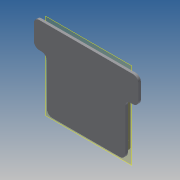
# Autodesk Inventor part: bottom plate cap
Saved by Autodesk Inventor 2013 (Build 170138000, 138)
## iProperties
Created: 2017-04-08
Part Number: bottom plate cap
Material: Generic
Document SubType Name: Modeling
Designer: employee
Density: 1 g/cm^3
Author: employee
Autodesk Inventor part; units mm, degrees
ref_plane "YZ Plane" through (0, 0, 0) normal (1, 0, 0) x (0, 1, 0)
ref_plane "XZ Plane" through (0, 0, 0) normal (0, 1, 0) x (-1, 0, 0)
ref_plane "XY Plane" through (0, 0, 0) normal (0, 0, 1) x (1, 0, 0)
ref_plane "Work Plane1" through (0, 0, 0) normal (0, 0, 1) x (1, 0, 0)
sketch "Sketch1" plane through (0, 0, 0) normal (0, 0, 1) x (1, 0, 0)
  line L0 (70, 65) -> (70, -65) projected
  arc A0 (65, -70) -> (70, -65) centre (65, -65) ccw projected
  line L1 (65, -70) -> (-65, -70) projected
  arc A1 (-70, -65) -> (-65, -70) centre (-65, -65) ccw projected
  line L2 (-70, -65) -> (-70, 65) projected
  arc A2 (-65, 70) -> (-70, 65) centre (-65, 65) ccw projected
  line L3 (-65, 70) -> (65, 70) projected
  arc A3 (70, 65) -> (65, 70) centre (65, 65) ccw projected
  arc A4 (-75, -65) -> (-65, -75) centre (-65, -65) ccw projected
  line L4 (-65, -75) -> (65, -75) projected
  arc A5 (65, -75) -> (75, -65) centre (65, -65) ccw projected
  line L5 (75, -65) -> (75, 65) projected
  arc A6 (75, 65) -> (65, 75) centre (65, 65) ccw projected
  line L6 (65, 75) -> (-65, 75) projected
  arc A7 (-65, 75) -> (-75, 65) centre (-65, 65) ccw projected
  line L7 (-75, 65) -> (-75, -65) projected
  line L8 (-65, 65) -> (-65, -65)
  line L9 (-65, -65) -> (65, -65)
  line L10 (65, -65) -> (65, 65)
  line L11 (65, 65) -> (-65, 65)
  point P0 (0, 0)
  dimension "d0" = 5
  constraints: 8 end point, 23 other
  measures "d0" distance between parallel lines of L8 L2
extrude "Extrusion1" add sketch "Sketch1" against normal blind 10 contours L0 A0 L1 A1 L2 A2 L3 A3
sketch "Sketch2" plane through (0, 0, 0) normal (0, 0, 1) x (1, 0, 0)
  line L0 (65, -65) -> (-65, -65) projected
  line L1 (70, 65) -> (70, -65) construction
  arc A0 (65, -70) -> (70, -65) centre (65, -65) ccw projected
  line L2 (65, -70) -> (-65, -70) projected
  arc A1 (-70, -65) -> (-65, -70) centre (-65, -65) ccw projected
  line L3 (-70, -65) -> (-70, 65) projected
  arc A2 (-65, 70) -> (-70, 65) centre (-65, 65) ccw projected
  line L4 (-65, 70) -> (65, 70) projected
  arc A3 (70, 65) -> (65, 70) centre (65, 65) ccw projected
  arc A4 (-75, -65) -> (-65, -75) centre (-65, -65) ccw projected
  line L5 (-65, -75) -> (65, -75) projected
  arc A5 (65, -75) -> (75, -65) centre (65, -65) ccw projected
  line L6 (75, -65) -> (75, 65) projected
  arc A6 (75, 65) -> (65, 75) centre (65, 65) ccw construction
  line L7 (65, 75) -> (-65, 75) projected
  arc A7 (-65, 75) -> (-75, 65) centre (-65, 65) ccw projected
  line L8 (-75, 65) -> (-75, -65) projected
  line L9 (-65, 75) -> (-90, 75)
  arc A8 (-90, 75) -> (-100, 65) centre (-90, 65) ccw
  line L10 (-100, 65) -> (-100, 35)
  arc A9 (-100, 35) -> (-90, 25) centre (-90, 35) ccw
  line L11 (-90, 25) -> (-85, 25)
  arc A10 (-75, 15) -> (-85, 25) centre (-85, 15) ccw
  line L12 (65, 75) -> (90, 75)
  arc A11 (100, 65) -> (90, 75) centre (90, 65) ccw
  line L13 (100, 65) -> (100, 35)
  arc A12 (90, 25) -> (100, 35) centre (90, 35) ccw
  line L14 (90, 25) -> (85, 25)
  line L15 (65, 75) -> (-65, 75)
  line L16 (-75, 15) -> (-75, -65)
  arc A13 (85, 25) -> (75, 15) centre (85, 15) ccw
  line L17 (75, 15) -> (75, -65)
  point P0 (0, 0)
  dimension "d3" = 25
  dimension "d4" = 50
  constraints: 20 tangent, 18 end point, 12 point on circle, 6 centre point, 6 equal radius, 4 perpendicular, 3 parallel, 2 collinear, 2 equal length, 2 point on line
  measures "d3" distance between parallel lines of L10 L8
  measures "d4" distance between parallel lines of L14 L12
extrude "Extrusion2" add sketch "Sketch2" along normal blind 5
sketch "Sketch3" plane through (0, 0, -10) normal (0, 0, -1) x (-1, 0, 0)
  line L0 (-70, 65) -> (-70, -65) projected
  arc A0 (-70, -65) -> (-65, -70) centre (-65, -65) ccw projected
  line L1 (-65, -70) -> (65, -70) projected
  arc A1 (65, -70) -> (70, -65) centre (65, -65) ccw projected
  line L2 (70, -65) -> (70, 65) projected
  arc A2 (70, 65) -> (65, 70) centre (65, 65) ccw projected
  line L3 (65, 70) -> (-65, 70) projected
  arc A3 (-65, 70) -> (-70, 65) centre (-65, 65) ccw projected
  line L4 (-69.5, -65) -> (-69.5, 65)
  arc A4 (-65, 69.5) -> (-69.5, 65) centre (-65, 65) ccw
  line L5 (-65, 69.5) -> (65, 69.5)
  arc A5 (69.5, 65) -> (65, 69.5) centre (65, 65) ccw
  line L6 (69.5, 65) -> (69.5, -65)
  arc A6 (65, -69.5) -> (69.5, -65) centre (65, -65) ccw
  line L7 (65, -69.5) -> (-65, -69.5)
  arc A7 (-69.5, -65) -> (-65, -69.5) centre (-65, -65) ccw
  point P0 (0, 0)
  dimension "d7" = 0.5
  constraints: 8 end point, 8 point on circle, 4 centre point, 7 other
  measures "d7" distance between parallel lines of L0 L4
extrude "Extrusion3" cut sketch "Sketch3" against normal up to surface (10 mm away)
sketch "Sketch4" plane through (-69.5, -65, -10) normal (-1, 0, 0) x (0, 0, 1)
  circle A0 centre (5, 115) radius 1.75 projected
  circle A1 centre (5, 15) radius 1.75 projected
  line L0 (-55.6, 130) -> (-55, 129.4) projected
  line L1 (-55, 129.4) -> (-15.8284, 129.4) projected
  arc A2 (-15.8284, 129.4) -> (-14.4142, 129.9858) centre (-15.8284, 131.4) ccw projected
  line L2 (-13.5858, 130.8142) -> (-14.4142, 129.9858) projected
  arc A3 (-13.5858, 130.8142) -> (-13, 132.2284) centre (-15, 132.2284) ccw projected
  line L3 (-13, 132.2284) -> (-13, 132.5) projected
  line L4 (-13, 132.5) -> (1, 132.5) projected
  line L5 (1, 130) -> (1, 132.5) projected
  line L6 (1, 130) -> (10, 130) projected
  line L7 (10, 0) -> (10, 130) projected
  line L8 (-65, 0) -> (10, 0) projected
  line L9 (-65, 130) -> (-65, 0) projected
  line L10 (-65, 130) -> (-55.6, 130) projected
  line L11 (-17.5711, 15) -> (-10.5, 7.9289) projected
  line L12 (-10.5, 7.9289) -> (-3.4289, 15) projected
  line L13 (-3.4289, 15) -> (-10.5, 22.0711) projected
  line L14 (-10.5, 22.0711) -> (-17.5711, 15) projected
  line L15 (-17.5711, 40) -> (-10.5, 32.9289) projected
  line L16 (-10.5, 32.9289) -> (-3.4289, 40) projected
  line L17 (-3.4289, 40) -> (-10.5, 47.0711) projected
  line L18 (-10.5, 47.0711) -> (-17.5711, 40) projected
  line L19 (-17.5711, 65) -> (-10.5, 57.9289) projected
  line L20 (-10.5, 57.9289) -> (-3.4289, 65) projected
  line L21 (-3.4289, 65) -> (-10.5, 72.0711) projected
  line L22 (-10.5, 72.0711) -> (-17.5711, 65) projected
  line L23 (-17.5711, 90) -> (-10.5, 82.9289) projected
  line L24 (-10.5, 82.9289) -> (-3.4289, 90) projected
  line L25 (-3.4289, 90) -> (-10.5, 97.0711) projected
  line L26 (-10.5, 97.0711) -> (-17.5711, 90) projected
  line L27 (-17.5711, 115) -> (-10.5, 107.9289) projected
  line L28 (-10.5, 107.9289) -> (-3.4289, 115) projected
  line L29 (-3.4289, 115) -> (-10.5, 122.0711) projected
  line L30 (-10.5, 122.0711) -> (-17.5711, 115) projected
  line L31 (-37.5711, 15) -> (-30.5, 7.9289) projected
  line L32 (-30.5, 7.9289) -> (-23.4289, 15) projected
  line L33 (-23.4289, 15) -> (-30.5, 22.0711) projected
  line L34 (-30.5, 22.0711) -> (-37.5711, 15) projected
  line L35 (-37.5711, 40) -> (-30.5, 32.9289) projected
  line L36 (-30.5, 32.9289) -> (-23.4289, 40) projected
  line L37 (-23.4289, 40) -> (-30.5, 47.0711) projected
  line L38 (-30.5, 47.0711) -> (-37.5711, 40) projected
  line L39 (-37.5711, 90) -> (-30.5, 82.9289) projected
  line L40 (-30.5, 82.9289) -> (-23.4289, 90) projected
  line L41 (-23.4289, 90) -> (-30.5, 97.0711) projected
  line L42 (-30.5, 97.0711) -> (-37.5711, 90) projected
  line L43 (-37.5711, 115) -> (-30.5, 107.9289) projected
  line L44 (-30.5, 107.9289) -> (-23.4289, 115) projected
  line L45 (-23.4289, 115) -> (-30.5, 122.0711) projected
  line L46 (-30.5, 122.0711) -> (-37.5711, 115) projected
  line L47 (-57.5711, 15) -> (-50.5, 7.9289) projected
  line L48 (-50.5, 7.9289) -> (-43.4289, 15) projected
  line L49 (-43.4289, 15) -> (-50.5, 22.0711) projected
  line L50 (-50.5, 22.0711) -> (-57.5711, 15) projected
  line L51 (-57.5711, 40) -> (-50.5, 32.9289) projected
  line L52 (-50.5, 32.9289) -> (-43.4289, 40) projected
  line L53 (-43.4289, 40) -> (-50.5, 47.0711) projected
  line L54 (-50.5, 47.0711) -> (-57.5711, 40) projected
  line L55 (-57.5711, 65) -> (-50.5, 57.9289) projected
  line L56 (-50.5, 57.9289) -> (-43.4289, 65) projected
  line L57 (-43.4289, 65) -> (-50.5, 72.0711) projected
  line L58 (-50.5, 72.0711) -> (-57.5711, 65) projected
  line L59 (-57.5711, 90) -> (-50.5, 82.9289) projected
  line L60 (-50.5, 82.9289) -> (-43.4289, 90) projected
  line L61 (-43.4289, 90) -> (-50.5, 97.0711) projected
  line L62 (-50.5, 97.0711) -> (-57.5711, 90) projected
  line L63 (-57.5711, 115) -> (-50.5, 107.9289) projected
  line L64 (-50.5, 107.9289) -> (-43.4289, 115) projected
  line L65 (-43.4289, 115) -> (-50.5, 122.0711) projected
  line L66 (-50.5, 122.0711) -> (-57.5711, 115) projected
  line L67 (-30.5, 72.0711) -> (-37.5711, 65) projected
  line L68 (-37.5711, 65) -> (-30.5, 57.9289) projected
  line L69 (-30.5, 57.9289) -> (-23.4289, 65) projected
  line L70 (-23.4289, 65) -> (-30.5, 72.0711) projected
  point P0 (10, 65)
extrude "Extrusion4" cut sketch "Sketch4" against normal through all contours A0 | A1
sketch "Sketch5" plane through (65, -65, -10) normal (-1, 0, 0) x (0, 0, 1)
  circle A0 centre (5, 115) radius 1.75 projected
  circle A1 centre (5, 15) radius 1.75 projected
  line L0 (5, 111.8246) -> (2.25, 113.4123)
  line L1 (2.25, 113.4123) -> (2.25, 116.5877)
  line L2 (2.25, 116.5877) -> (5, 118.1754)
  line L3 (5, 118.1754) -> (7.75, 116.5877)
  line L4 (7.75, 116.5877) -> (7.75, 113.4123)
  line L5 (7.75, 113.4123) -> (5, 111.8246)
  line L6 (5, 18.1754) -> (7.75, 16.5877)
  line L7 (7.75, 16.5877) -> (7.75, 13.4123)
  line L8 (7.75, 13.4123) -> (5, 11.8246)
  line L9 (5, 11.8246) -> (2.25, 13.4123)
  line L10 (2.25, 13.4123) -> (2.25, 16.5877)
  line L11 (2.25, 16.5877) -> (5, 18.1754)
  point P0 (10, 65)
  dimension "d12" = 5.5
  constraints: 24 end point, 2 coincident, 2 vertical, 1 collinear, 26 other
  measures "d12" distance between parallel lines of L4 L1
extrude "Extrusion5" cut sketch "Sketch5" against normal blind 3
mirror "Mirror1" about plane through (0, 0, 0) normal (1, 0, 0) of "Extrusion5"
sketch "Sketch6" plane through (0, 0, -10) normal (0, 0, -1) x (-1, 0, 0)
  line L0 (-65, 65) -> (65, 65) projected
  line L1 (-87.6813, 89.7845) -> (86.894, 89.7845)
  line L2 (86.894, 89.7845) -> (86.894, 60)
  line L3 (86.894, 60) -> (-87.6813, 60)
  line L4 (-87.6813, 60) -> (-87.6813, 89.7845)
  line L5 (-90, 75) -> (90, 75) projected
  point P0 (0, 0)
  dimension "d15" = 15
  constraints: 8 end point, 3 parallel, 1 perpendicular
  measures "d15" distance between parallel lines of L3 L5
extrude "Extrusion6" cut sketch "Sketch6" against normal blind 5
body "Solid1"
